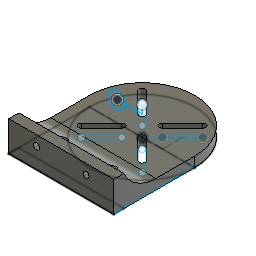
support (Autodesk Fusion 360 design; units mm, degrees)
Autodesk Fusion 360 part; units mm, degrees
note: some values were not read from the file. Set by a fixed rule: which sketch regions a step uses.
sketch "Esquisse1" plane through (0, 0, 0) normal (0, 1, 0) x (1, 0, 0)
  circle A0 centre (0, 0) radius 26
  line L0 (0, 0) -> (-26, 0) construction
  line L1 (0, 0) -> (26, 0) construction
  line L2 (-26, 0) -> (26, 0)
  line L3 (26, 0) -> (26, -40)
  line L4 (26, -40) -> (-26, -40)
  line L5 (-26, -40) -> (-26, 0)
  line L6 (-26, -40) -> (26, -40)
  line L7 (26, -40) -> (26, -35)
  line L8 (26, -35) -> (-26, -35)
  line L9 (-26, -35) -> (-26, -40)
  line L10 (0, 0) -> (15, 15)
  line L11 (13.9393, 16.0607) -> (3.9393, 6.0607)
  arc A1 (3.9393, 6.0607) -> (6.0607, 3.9393) centre (5, 5) ccw
  line L12 (6.0607, 3.9393) -> (16.0607, 13.9393)
  arc A2 (16.0607, 13.9393) -> (13.9393, 16.0607) centre (15, 15) ccw
  line L13 (15, 15) -> (5, 5) construction
  line L14 (0, 0) -> (10, 0) construction
  line L15 (10, 0) -> (10, 10) construction
  line L16 (-3.9393, 6.0607) -> (-13.9393, 16.0607)
  arc A3 (-6.0607, 3.9393) -> (-3.9393, 6.0607) centre (-5, 5) ccw
  line L17 (-16.0607, 13.9393) -> (-6.0607, 3.9393)
  arc A4 (-13.9393, 16.0607) -> (-16.0607, 13.9393) centre (-15, 15) ccw
  line L18 (-6.0607, -3.9393) -> (-16.0607, -13.9393)
  arc A5 (-3.9393, -6.0607) -> (-6.0607, -3.9393) centre (-5, -5) ccw
  line L19 (-13.9393, -16.0607) -> (-3.9393, -6.0607)
  arc A6 (-16.0607, -13.9393) -> (-13.9393, -16.0607) centre (-15, -15) ccw
  line L20 (3.9393, -6.0607) -> (13.9393, -16.0607)
  arc A7 (6.0607, -3.9393) -> (3.9393, -6.0607) centre (5, -5) ccw
  line L21 (16.0607, -13.9393) -> (6.0607, -3.9393)
  arc A8 (13.9393, -16.0607) -> (16.0607, -13.9393) centre (15, -15) ccw
  dimension "d1" = 52
  dimension "d2" = 40
  dimension "d3" = 5
  dimension "d4" = 3
  dimension "d5" = 10
  dimension "d7" = 360
  constraint coincident A0.centre L0.start
  constraint coincident A0 L0.end
  constraint horizontal L0
  constraint coincident A0 L1.end
  constraint parallel L0 L1
  constraint horizontal L2
  constraint vertical L3
  constraint horizontal L4
  constraint vertical L5
  constraint horizontal L6
  constraint vertical L7
  constraint horizontal L8
  constraint vertical L9
  constraint coincident L3 L7.end
  constraint tangent L11 A1
  constraint tangent A1 L12
  constraint parallel L11 L12
  constraint tangent L12 A2
  constraint tangent L11 A2
  constraint coincident L10 A1.centre
  constraint parallel L10 L13
  constraint coincident L10.end A2.centre
  constraint parallel L1 L14
  constraint midpoint L13 L15.end
  constraint perpendicular L14 L15
  measures "d1" diameter of A0
  measures "d2" distance of L0.end L4.end
  measures "d3" distance of L4.end L8.end
  measures "d4" diameter of A1
  measures "d5" distance of A0.centre L14.end
extrude "Extrusion1" add sketch "Esquisse1" along normal blind 5 contours A0 L2 | A0 L3 L5 L8 | A0 L2
extrude "Extrusion2" add sketch "Esquisse1" along normal blind 15 contours L3 L4 L5 L6 L7 L8 L9
fillet "Congé1" radius 17.5 1 edges at (0, 5, 35)
sketch "Esquisse2" plane through (0, 0, 0) normal (0, 0, 1) x (1, 0, 0)
  line L0 (0, 10) -> (-12.25, 10)
  circle A0 centre (-12.25, 10) radius 1.5
  circle A1 centre (-12.25, 10) radius 4
  line L1 (0, 10) -> (0, 14)
  dimension "d14" = 12.25
  dimension "d15" = 3
  dimension "d16" = 8
  constraint horizontal L0
  constraint coincident L0.end A0.centre
  constraint concentric A0 A1
  constraint perpendicular L0 L1
  measures "d14" distance of L0.start L0.end
  measures "d15" diameter of A0
  measures "d16" diameter of A1
extrude "Extrusion3" cut sketch "Esquisse2" along normal blind 73 contours A0
extrude "Extrusion4" cut sketch "Esquisse2" along normal blind 35
mirror "Symétrie miroir1" about plane through (0, 0, 0) normal (1, 0, 0) of "Extrusion4"
mirror "Symétrie miroir2" about plane through (0, 0, 0) normal (1, 0, 0) of "Extrusion3"
equation "d2 = 66 mm - 26 mm"
